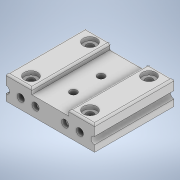
# Autodesk Inventor part: slidesmount
Saved by Autodesk Inventor 2020 (Build 240168000, 168)
## iProperties
Created: 2019-12-18
Part Number: slidesmount
Material: Generic
Document SubType Name: Modeling
Designer: xj82b
Density: 1 g/cm^3
Appearance: Default
Author: xj82b
Autodesk Inventor part; units mm, degrees
ref_plane "YZ Plane" through (0, 0, 0) normal (1, 0, 0) x (0, 1, 0)
ref_plane "XZ Plane" through (0, 0, 0) normal (0, 1, 0) x (-1, 0, 0)
ref_plane "XY Plane" through (0, 0, 0) normal (0, 0, 1) x (1, 0, 0)
sketch "Sketch1" plane through (0, 0, 0) normal (0, 1, 0) x (-1, 0, 0)
  line L0 (0, 0) -> (-48, 0)
  line L1 (-48, 0) -> (-48, -43)
  line L2 (-48, -43) -> (0, -43)
  line L3 (0, -43) -> (0, 0)
  circle A0 centre (-24, -27.5) radius 1.95
  circle A1 centre (-24, -12.5) radius 1.95
  circle A2 centre (-8, -5.5) radius 1.95
  circle A3 centre (-40, -5.5) radius 1.95
  circle A4 centre (-40, -37.5) radius 1.95
  circle A5 centre (-8, -37.5) radius 1.95
  point P0 (-24, -43)
  dimension "d0" = 48
  dimension "d1" = 43
  dimension "d2" = 3.9
  dimension "d3" = 3.9
  dimension "d4" = 15
  dimension "d5" = 12.5
  dimension "d6" = 3.9
  dimension "d7" = 3.9
  dimension "d8" = 3.9
  dimension "d9" = 3.9
  dimension "d10" = 32
  dimension "d11" = 8
  dimension "d12" = 5.5
  dimension "d13" = 5.5
  constraints: 8 end point, 6 centre point, 4 vertical alignment, 2 horizontal alignment, 2 parallel, 1 horizontal, 1 midpoint, 1 perpendicular
  measures "d0" distance of L2.end L1.end
  measures "d1" distance of L1.end L0.end
  measures "d2" diameter of A0
  measures "d3" diameter of A1
  measures "d4" distance of A1.centre A0.centre
  measures "d5" distance from line of L0 A1.centre
  measures "d6" diameter of A2
  measures "d7" diameter of A3
  measures "d8" diameter of A4
  measures "d9" diameter of A5
  measures "d10" distance of A2.centre A3.centre
  measures "d11" distance from line of L3 A2.centre
  measures "d12" distance from line of L0 A2.centre
  measures "d13" distance from line of L2 A5.centre
extrude "Extrusion1" add sketch "Sketch1" along normal blind 15
sketch "Sketch2" plane through (0, 15, 0) normal (0, 1, 0) x (1, 0, 0)
  line L0 (14, 49.9518) -> (34, 49.9518)
  line L1 (34, 49.9518) -> (34, -4.9916)
  line L2 (34, -4.9916) -> (14, -4.9916)
  line L3 (14, -4.9916) -> (14, 49.9518)
  line L4 (48, 43) -> (0, 43) projected
  point P0 (0, 0)
  point P1 (24, 49.9518)
  point P2 (24, 43)
  dimension "d16" = 20
  constraints: 8 end point, 2 midpoint, 2 parallel, 1 horizontal, 1 perpendicular, 1 vertical alignment
  measures "d16" distance of L0.start L0.end
extrude "Extrusion2" cut sketch "Sketch2" against normal blind 5
sketch "Sketch3" plane through (48, 0, -43) normal (0, 0, -1) x (-1, 0, 0)
  circle A0 centre (16, 5.5) radius 1.95
  circle A1 centre (24, 5.5) radius 1.95
  circle A2 centre (32, 5.5) radius 1.95
  line L0 (34, 10) -> (14, 10) projected
  line L1 (0, 0) -> (48, 0) projected
  circle A3 centre (8, 5.5) radius 1.95
  circle A4 centre (40, 5.5) radius 1.95
  circle A5 centre (0, 5.5) radius 1.95
  circle A6 centre (48, 5.5) radius 1.95
  point P0 (24, 10)
  dimension "d19" = 3.9
  dimension "d20" = 3.9
  dimension "d21" = 3.9
  dimension "d22" = 8
  dimension "d23" = 8
  dimension "d24" = 5.5
  dimension "d25" = 3.9
  dimension "d26" = 3.9
  dimension "d27" = 8
  dimension "d28" = 8
  dimension "d29" = 3.9
  dimension "d30" = 3.9
  dimension "d31" = 8
  dimension "d32" = 8
  constraints: 7 centre point, 6 horizontal alignment, 1 midpoint, 1 vertical alignment
  measures "d19" diameter of A0
  measures "d20" diameter of A1
  measures "d21" diameter of A2
  measures "d22" distance of A1.centre A2.centre
  measures "d23" distance of A0.centre A1.centre
  measures "d24" distance from line of L1 A1.centre
  measures "d25" diameter of A3
  measures "d26" diameter of A4
  measures "d27" distance of A2.centre A4.centre
  measures "d28" distance of A3.centre A0.centre
  measures "d29" diameter of A5
  measures "d30" diameter of A6
  measures "d31" distance of A4.centre A6.centre
  measures "d32" distance of A5.centre A3.centre
extrude "Extrusion3" cut sketch "Sketch3" against normal through all contours A0 | A2 | A3 | A4 | A5 | A6
sketch "Sketch4" plane through (0, 0, 0) normal (0, -1, 0) x (1, 0, 0)
  circle A0 centre (16, -5.5) radius 3.75
  circle A1 centre (16, -37.5) radius 3.75
  circle A2 centre (32, -37.5) radius 3.75
  circle A3 centre (32, -5.5) radius 3.75
  line L0 (0, 0) -> (48, 0) projected
  circle A4 centre (40, -5.5) radius 1.95 projected
  dimension "d35" = 7.5
  dimension "d36" = 7.5
  dimension "d37" = 7.5
  dimension "d38" = 7.5
  dimension "d39" = 16
  dimension "d40" = 5.5
  dimension "d41" = 8
  dimension "d42" = 32
  constraints: 4 centre point, 2 horizontal alignment, 2 vertical alignment
  measures "d35" diameter of A0
  measures "d36" diameter of A1
  measures "d37" diameter of A2
  measures "d38" diameter of A3
  measures "d39" distance of A2.centre A1.centre
  measures "d40" distance from line of L0 A3.centre
  measures "d41" distance of A4.centre A3.centre
  measures "d42" distance of A0.centre A1.centre
extrude "Extrusion4" cut sketch "Sketch4" against normal blind 5 contours A0 | A1 | A2 | A3
fillet "Fillet1" radius 1 11 edges at (14, 15, -21.5) (34, 15, -21.5) (0, 15, -21.5) (48, 15, -21.5) (7, 15, -43) (41, 15, -43) (7, 15, 0) (41, 15, 0) (34, 12.5, -43) (14, 12.5, -43) (24, 10, -43)
sketch "Sketch5" plane through (0, 15, 0) normal (0, 1, 0) x (1, 0, 0)
  circle A0 centre (8, 5.5) radius 3.65
  circle A1 centre (40, 5.5) radius 3.65
  circle A2 centre (8, 37.5) radius 3.65
  circle A3 centre (40, 37.5) radius 3.65
  circle A4 centre (40, 37.5) radius 1.95 projected
  circle A5 centre (40, 5.5) radius 1.95 projected
  circle A6 centre (8, 37.5) radius 1.95 projected
  point P0 (0, 0)
  dimension "d46" = 7.3
  dimension "d47" = 7.3
  dimension "d48" = 7.3
  dimension "d49" = 7.3
  constraints: 4 centre point, 3 concentric, 2 horizontal alignment, 2 vertical alignment
  measures "d46" diameter of A0
  measures "d47" diameter of A1
  measures "d48" diameter of A2
  measures "d49" diameter of A3
extrude "Extrusion5" cut sketch "Sketch5" against normal blind 4
sketch "Sketch6" plane through (0, 0, 0) normal (0, -1, 0) x (1, 0, 0)
  line L0 (21.8927, -23.85) -> (26.1073, -23.85)
  line L1 (26.1073, -23.85) -> (28.2147, -27.5)
  line L2 (28.2147, -27.5) -> (26.1073, -31.15)
  line L3 (26.1073, -31.15) -> (21.8927, -31.15)
  line L4 (21.8927, -31.15) -> (19.7853, -27.5)
  line L5 (19.7853, -27.5) -> (21.8927, -23.85)
  line L6 (48, -43) -> (0, -43) projected
  line L7 (48, 0) -> (48, -43) projected
  line L8 (0, 0) -> (48, 0) projected
  line L9 (26.1073, -16.15) -> (21.8927, -16.15)
  line L10 (21.8927, -16.15) -> (19.7853, -12.5)
  line L11 (19.7853, -12.5) -> (21.8927, -8.85)
  line L12 (21.8927, -8.85) -> (26.1073, -8.85)
  line L13 (26.1073, -8.85) -> (28.2147, -12.5)
  line L14 (28.2147, -12.5) -> (26.1073, -16.15)
  point P0 (24, -27.5)
  point P1 (24, -12.5)
  dimension "d52" = 7.3
  dimension "d53" = 24
  dimension "d55" = 27.5
  dimension "d56" = 7.3
  dimension "d57" = 12.5
  dimension "d58" = 24
  constraints: 24 end point, 2 parallel, 26 other
  measures "d52" distance between parallel lines of L0 L3
  measures "d53" distance from line of L7 point (24, -27.5)
  measures "d55" distance from line of L8 point (24, -27.5)
  measures "d56" distance between parallel lines of L12 L9
  measures "d57" distance from line of L8 point (24, -12.5)
  measures "d58" distance from line of L7 point (24, -12.5)
extrude "Extrusion6" cut sketch "Sketch6" against normal blind 5
sketch "Sketch7" plane through (0, 15, 0) normal (0, 1, 0) x (1, 0, 0)
  line L0 (-2.812, 43.9982) -> (53.4288, 43.9982)
  line L1 (53.4288, 43.9982) -> (53.4288, -3.3264)
  line L2 (53.4288, -3.3264) -> (-2.812, -3.3264)
  line L3 (-2.812, -3.3264) -> (-2.812, 43.9982)
  point P0 (0, 0)
  constraints: 8 end point, 2 parallel, 1 horizontal, 1 perpendicular
extrude "Extrusion7" cut sketch "Sketch7" against normal blind 2
fillet "Fillet2" radius 1 10 edges at (13.7071, 13, -42.7071) (6.5, 13, -43) (14, 13, -21) (34.2929, 13, -42.7071) (41.5, 13, -43) (34, 13, -21) (41, 13, 0) (48, 13, -21.5) (0, 13, -21.5) (7, 13, 0)
body "Solid1"
